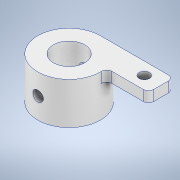
# Autodesk Inventor part: ShaftGuide
Saved by Autodesk Inventor 2022.2 (Build 262287030, 287C)
## iProperties
Created: 2023-03-20
Part Number: ShaftGuide
Material: Aluminum 6061
Document SubType Name: Modeling
Designer: jak27277
Density: 2.7 g/cm^3
Appearance: Aluminum - Flat
Author: jak27277
Autodesk Inventor part; units mm, degrees
ref_plane "YZ Plane" through (0, 0, 0) normal (1, 0, 0) x (0, 1, 0)
ref_plane "XZ Plane" through (0, 0, 0) normal (0, 1, 0) x (-1, 0, 0)
ref_plane "XY Plane" through (0, 0, 0) normal (0, 0, 1) x (1, 0, 0)
sketch "Sketch1" plane through (0, 0, 0) normal (0, 1, 0) x (-1, 0, 0)
  circle A0 centre (0, 0) radius 19.05
  circle A1 centre (0, 0) radius 9.525
  dimension "d0" = 38.1
  dimension "d1" = 19.05
  constraints: 2 centre point, 2 coincident
  measures "d0" diameter of A0
  measures "d1" diameter of A1
extrude "Extrusion1" add sketch "Sketch1" along normal blind 25.4
sketch "Sketch2" plane through (0, 25.4, 0) normal (0, 1, 0) x (1, 0, 0)
  circle A0 centre (0, 0) radius 19.05 projected
  line L0 (0, 19.05) -> (44.45, 19.05)
  line L1 (44.45, 19.05) -> (44.45, 3.81)
  line L2 (44.45, 3.81) -> (18.6651, 3.81)
  line L3 (44.45, 11.43) -> (15.24, 11.43)
  circle A1 centre (34.29, 11.43) radius 3.175
  dimension "d4" = 44.45
  dimension "d5" = 15.24
  dimension "d6" = 6.35
  dimension "d7" = 10.16
  constraints: 8 end point, 3 point on circle, 2 horizontal, 2 perpendicular, 1 centre point, 1 midpoint, 1 point on line, 1 tangent
  measures "d4" distance of L0.start L0.end
  measures "d5" distance of L0.end L1.end
  measures "d6" diameter of A1
  measures "d7" distance from line of L1 A1.centre
extrude "Extrusion2" add sketch "Sketch2" against normal blind 6.35 contours A0 L3 A1 L1 L2 | L0 L1 L3 A1 A0
fillet "Fillet1" radius 3.175 3 edges at (18.6651, 22.225, -3.81) (44.45, 22.225, -3.81) (44.45, 22.225, -19.05)
sketch "Sketch3" plane through (0, 19.05, -19.05) normal (0, 0, -1) x (-1, 0, 0)
  circle A0 centre (0, -6.35) radius 3.175
  line L0 (19.05, -19.05) -> (-19.05, -19.05) projected
  point P0 (0, -19.05)
  point P1 (0, -19.05)
  dimension "d11" = 12.7
  dimension "d12" = 6.35
  constraints: 1 centre point, 1 midpoint, 1 vertical alignment
  measures "d11" distance from line of A0.centre L0
  measures "d12" diameter of A0
extrude "Extrusion3" cut sketch "Sketch3" against normal through all
body "Solid1"
